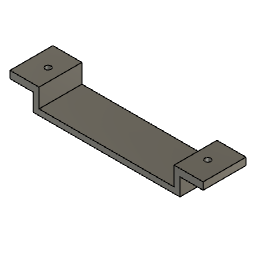
bracket v3 (Autodesk Fusion 360 design; units mm, degrees)
Autodesk Fusion 360 part; units mm, degrees
note: some values were not read from the file. Set by a fixed rule: which face or edge a step refers to.
sketch "Sketch1" plane through (0, 0, 0) normal (0, 0, 1) x (1, 0, 0)
  line L0 (50.5, -44.75) -> (-50.5, -44.75)
  line L1 (-50.5, -44.75) -> (-50.5, 44.75)
  line L2 (-50.5, 44.75) -> (50.5, 44.75)
  line L3 (50.5, 44.75) -> (50.5, -44.75)
  line L4 (50.5, -44.75) -> (-50.5, 44.75) construction
  line L5 (-50.5, -44.75) -> (50.5, 44.75) construction
  dimension "d1" = 101
  dimension "d2" = 89.5
  constraint horizontal L0
  constraint perpendicular L0 L1
  constraint parallel L0 L2
  constraint parallel L1 L3
  constraint coincident L4 origin
  constraint coincident L5 origin
  measures "d1" distance of L1.end L2.end
  measures "d2" distance of L0.end L1.end
extrude "Extrude1" add sketch "Sketch1" along normal blind 12
shell "Shell1" thickness 4 removed faces 1 at (-16.8333, 14.9167, 12)
extrude "Extrude2" cut 1 faces at (15.5, 40.75, 6.6667) along direction (0, -1, 0) up to surface (85.5 mm away) and the other way up to surface (4 mm away)
sketch "Sketch3" plane through (0, 0, 12) normal (0, 0, 1) x (-1, 0, 0)
  line L0 (46.5, 44.75) -> (46.5, -44.75)
  line L1 (46.5, -44.75) -> (50.5, -44.75)
  line L2 (50.5, -44.75) -> (50.5, 44.75)
  line L3 (50.5, 44.75) -> (46.5, 44.75)
  line L4 (46.5, -44.75) -> (66.5, -44.75)
  line L5 (66.5, -44.75) -> (66.5, 44.75)
  line L6 (66.5, 44.75) -> (46.5, 44.75)
  line L7 (46.5, 44.75) -> (46.5, -44.75)
  line L8 (0, -2.5) -> (0, -20)
  line L9 (-46.5, -44.75) -> (-66.5, -44.75)
  line L10 (-66.5, -44.75) -> (-66.5, 44.75)
  line L11 (-46.5, 44.75) -> (-46.5, -44.75)
  line L12 (-66.5, 44.75) -> (-46.5, 44.75)
  line L13 (0, 0) -> (55, 0) construction
  circle A0 centre (55, 0) radius 2
  circle A1 centre (-55, 0) radius 2
  dimension "d15" = 89.5
  dimension "d16" = 20
  dimension "d21" = 55
  dimension "d22" = 4
  constraint perpendicular L4 L5
  constraint parallel L4 L6
  constraint parallel L5 L7
  constraint perpendicular L2 L4
  constraint coincident L0.end L1.start
  constraint symmetric L0.end L8 L9.start
  constraint symmetric L4.end L8 L9.end
  constraint symmetric L5.end L8 L10.end
  constraint symmetric L0.start L8 L11.start
  constraint coincident L13.start origin
  constraint perpendicular L2 L13
  constraint coincident L13.end A0.centre
  constraint symmetric L8 A0 A1
  measures "d15" distance of L4.end L5.end
  measures "d16" distance of L5.end L0.start
  measures "d21" distance of L13.start L13.end
  measures "d22" diameter of A0
extrude "Extrude4" add sketch "Sketch3" along normal blind 5
move_face "OffsetFaces1" offset -30 1 faces at (54.5, -44.75, 15.3333)
move_face "OffsetFaces2" offset -30 1 faces at (54.5, 44.75, 15.3333)
